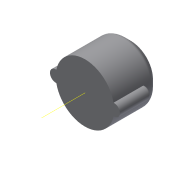
# Autodesk Inventor part: case
Saved by Autodesk Inventor 2014 (Build 180170000, 170)
## iProperties
Created: 2014-01-08
Part Number: case
Material: Generisch
Document SubType Name: Modeling
Designer: Felix
Density: 1 g/cm^3
Appearance: Vorgabe
Author: Felix
Autodesk Inventor part; units mm, degrees
ref_plane "YZ Plane" through (0, 0, 0) normal (1, 0, 0) x (0, 1, 0)
ref_plane "XZ Plane" through (0, 0, 0) normal (0, 1, 0) x (-1, 0, 0)
ref_plane "XY Plane" through (0, 0, 0) normal (0, 0, 1) x (1, 0, 0)
sketch "Skizze1" plane through (0, 0, 0) normal (0, 1, 0) x (-1, 0, 0)
  circle A0 centre (0, 0) radius 7.5
  circle A1 centre (7.5, 0) radius 1.5
  circle A2 centre (-7.5, 0) radius 1.5
  dimension "d0" = 15
  dimension "d1" = 3
  dimension "d2" = 3
  constraints: 3 centre point, 2 point on circle, 1 coincident
  measures "d0" diameter of A0
  measures "d1" diameter of A1
  measures "d2" diameter of A2
extrude "Extrusion1" add sketch "Skizze1" along normal blind 12 contours A0 A1 | A1 A0 A2 | A2 A0 picked at (7.0094, -0.2882) picked at (-6.9889, 0)
sketch "Skizze2" plane through (0, 0, 0) normal (0, -1, 0) x (1, 0, 0)
  circle A0 centre (0, 0) radius 7.5 projected
  circle A1 centre (7.5, 0) radius 1.5
  circle A2 centre (-7.5, 0) radius 1.5
  dimension "d5" = 3
  dimension "d6" = 3
  constraints: 2 centre point, 2 point on circle
  measures "d5" diameter of A1
  measures "d6" diameter of A2
extrude "Extrusion2" add sketch "Skizze2" against normal blind 8 contours A0 A1 | A0 A1 | A2 A0 | A0 A2
chamfer "Fase1" distance 2 angle 45 1 edges at (7.5, 12, 0)
fillet "Rundung1" radius 1 2 edges at (7.5, 10, 0) (5.5, 12, 0)
fillet "Rundung2" radius 0.5 2 edges at (9, 8, 0) (-9, 8, 0)
